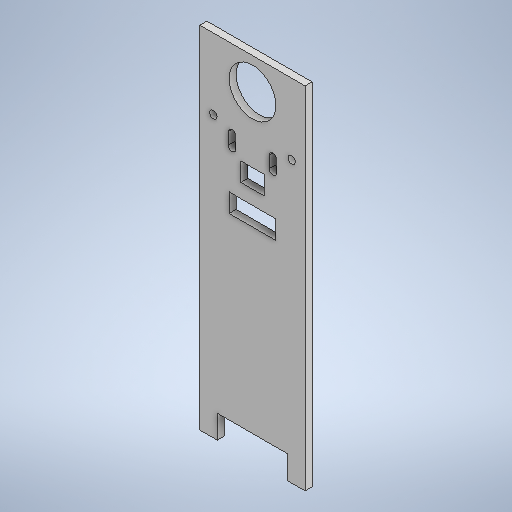
# Autodesk Inventor part: DC Motor Fixing Wall
Saved by Autodesk Inventor 2025.4 (Build 294407000, 407)
## iProperties
Created: 2026-05-09
Part Number: DC Motor Fixing Wall
Material: Generic
Document SubType Name: Sheet Metal
Designer: lenovo
Density: 1 g/cm^3
Sheet Metal Rule: Default_mm
Appearance: Default
Author: lenovo
Autodesk Inventor part; units mm, degrees
ref_plane "YZ Plane" through (0, 0, 0) normal (1, 0, 0) x (0, 1, 0)
ref_plane "XZ Plane" through (0, 0, 0) normal (0, 1, 0) x (-1, 0, 0)
ref_plane "XY Plane" through (0, 0, 0) normal (0, 0, 1) x (1, 0, 0)
sketch "Sketch1" plane through (0, 0, 0) normal (0, 0, 1) x (1, 0, 0)
  line L0 (-22.5, -75) -> (22.5, -75)
  line L1 (22.5, -75) -> (22.5, 75)
  line L2 (22.5, 75) -> (-22.5, 75)
  line L3 (-22.5, 75) -> (-22.5, -75)
  line L4 (-22.5, -75) -> (22.5, 75) construction
  line L5 (22.5, -75) -> (-22.5, 75) construction
  circle A0 centre (0, 61.5) radius 10
  circle A1 centre (16.75, 44.75) radius 1.6
  line L6 (0, 75) -> (0, -75)
  circle A2 centre (8.75, 41.65) radius 1.6
  circle A3 centre (-16.75, 44.75) radius 1.6
  circle A4 centre (-8.75, 41.65) radius 1.6
  line L7 (-15.04, -75) -> (15.04, -75)
  line L8 (15.04, -75) -> (15.04, -65)
  line L9 (15.04, -65) -> (-15.04, -65)
  line L10 (-15.04, -65) -> (-15.04, -75)
  line L11 (-5, 33.5) -> (5, 33.5)
  line L12 (5, 33.5) -> (5, 25.5)
  line L13 (5, 25.5) -> (-5, 25.5)
  line L14 (-5, 25.5) -> (-5, 33.5)
  line L15 (-5, 33.5) -> (5, 25.5) construction
  line L16 (5, 33.5) -> (-5, 25.5) construction
  line L17 (-10, 19.5) -> (10, 19.5)
  line L18 (10, 19.5) -> (10, 11.5)
  line L19 (10, 11.5) -> (-10, 11.5)
  line L20 (-10, 11.5) -> (-10, 19.5)
  line L21 (-10, 19.5) -> (10, 11.5) construction
  line L22 (10, 19.5) -> (-10, 11.5) construction
  line L23 (8.75, 41.65) -> (8.75, 36.65) construction
  line L24 (7.15, 41.65) -> (7.15, 36.65)
  line L25 (10.35, 36.65) -> (10.35, 41.65)
  arc A5 (10.35, 41.65) -> (7.15, 41.65) centre (8.75, 41.65) ccw
  arc A6 (7.15, 36.65) -> (10.35, 36.65) centre (8.75, 36.65) ccw
  line L26 (-7.15, 41.65) -> (-7.15, 36.65)
  line L27 (-10.35, 36.65) -> (-10.35, 41.65)
  arc A7 (-10.35, 36.65) -> (-7.15, 36.65) centre (-8.75, 36.65) ccw
  point P0 (0, 0)
  point P1 (0, -65)
  point P2 (0, 29.5)
  point P3 (0, 33.5)
  point P4 (0, 15.5)
  point P5 (8.75, 39.15)
  point P6 (10.35, 41.65)
  point P7 (-7.15, 41.65)
  dimension "d0" = 20
  dimension "d1" = 136.5
  dimension "d2" = 150
  dimension "d3" = 45
  dimension "d4" = 3.2
  dimension "d5" = 119.75
  dimension "d6" = 33.5
  dimension "d7" = 3.2
  dimension "d8" = 116.65
  dimension "d9" = 17.5
  dimension "d10" = 30.08
  dimension "d11" = 10
  dimension "d12" = 28
  dimension "d13" = 8
  dimension "d14" = 10
  dimension "d15" = 46
  dimension "d16" = 8
  dimension "d17" = 20
  dimension "d19" = 5
  measures "d0" diameter of A0
  measures "d1" distance from line of L0 A0.centre
  measures "d2" distance of L2.end L0.start
  measures "d3" distance of L0.start L0.end
  measures "d4" diameter of A1
  measures "d5" distance from line of L0 A1.centre
  measures "d6" diameter of A1.centre L6
  measures "d7" diameter of A2
  measures "d8" distance from line of L23.start L0
  measures "d9" diameter of L23.start L6
  measures "d10" distance of L8.end L9.end
  measures "d11" distance of L7.end L8.end
  measures "d12" distance of A0.centre point (0, 33.5)
  measures "d13" distance of L13.end L11.start
  measures "d14" distance of L12.end L13.end
  measures "d15" distance of point (0, 15.5) A0.centre
  measures "d16" distance of L17.end L18.end
  measures "d17" distance of L18.end L19.end
  measures "d19" distance of L23.start L23.end
extrude "Plate1" add sketch "Sketch1" along normal blind 3 contours L3 L2 L6 A0 L11 L14 L13 L17 L20 L19 L9 L10 L0 | L2 L1 L0 L8 L9 L6 L19 L18 L17 L13 L12 L11 A0
equation "\"d18\" = Thickness"
equation "\"BendRadius\" = Thickness"
equation "\"BendReliefWidth\" = Thickness"
equation "\"BendReliefDepth\" = 0.5 * Thickness"
equation "\"CornerReliefSize\" = 4 * Thickness"
equation "\"MinimumRemnant\" = 2 * Thickness"
equation "\"TransitionRadius\" = BendRadius"
equation "\"JacobiRadiusSize\" = BendRadius"
equation "\"GapSize\" = Thickness"
equation "\"Thickness\" = 3"
body "Solid1"
